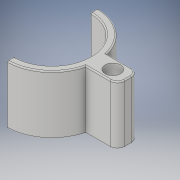
# Autodesk Inventor part: Camera Clip
Saved by Autodesk Inventor 2019.4 (Build 234330000, 330)
## iProperties
Created: 2021-02-04
Part Number: Camera Clip
Material: Generic
Document SubType Name: Modeling
Designer: caleb
Density: 1 g/cm^3
Appearance: Default
Author: caleb
Autodesk Inventor part; units mm, degrees
ref_plane "YZ Plane" through (0, 0, 0) normal (1, 0, 0) x (0, 1, 0)
ref_plane "XZ Plane" through (0, 0, 0) normal (0, 1, 0) x (-1, 0, 0)
ref_plane "XY Plane" through (0, 0, 0) normal (0, 0, 1) x (1, 0, 0)
sketch "Sketch1" plane through (0, 0, 0) normal (0, 1, 0) x (-1, 0, 0)
  circle A0 centre (0, 0) radius 16.51
  circle A1 centre (0, 0) radius 19.685
  line L0 (0, 19.685) -> (0, -19.685)
  line L1 (-32.9172, 4.594) -> (-17.9063, 4.594)
  line L2 (-17.9063, 4.594) -> (-17.9063, -4.594)
  line L3 (-17.9063, -4.594) -> (-32.9172, -4.594)
  line L4 (-32.9172, -4.594) -> (-32.9172, 4.594)
  line L5 (-32.9172, 4.594) -> (-17.9063, -4.594) construction
  line L6 (-17.9063, 4.594) -> (-32.9172, -4.594) construction
  point P0 (-25.4118, 0)
  dimension "d0" = 33.02
  dimension "d1" = 39.37
  constraints: 14 end point, 2 centre point, 2 coincident, 2 midpoint, 2 parallel, 2 point on circle, 1 horizontal, 1 perpendicular, 1 vertical
  measures "d0" diameter of A0
  measures "d1" diameter of A1
extrude "Extrusion1" add sketch "Sketch1" along normal blind 25.4
extrude "Extrusion2" cut sketch "Sketch1" along normal blind 25.4 contours A0 L0 | L0 A0
extrude "Extrusion3" cut sketch "Sketch1" along normal blind 25.4 contours A0 L0 | A0 L0 A1 picked at (8.9586, -4.4939)
sketch "Sketch2" plane through (0, 25.4, 0) normal (0, 1, 0) x (1, 0, 0)
  point P0 (0, 0)
  point P1 (26.3547, 0)
hole "Hole1" at (26.3547, 25.4, 0) direction (0, -1, 0) diameter 6.7564 end through all clearance for "Flat Head Machine Screw (82)" size "1/4" standard "Ansi Unified Screw Threads"
fillet "Fillet1" radius 3.175 2 edges at (32.9172, 12.7, -4.594) (32.9172, 12.7, 4.594)
fillet "Fillet2" radius 0.508 24 edges at (12.1874, 25.4, -15.4585) (16.51, 25.4, 0) (12.1874, 25.4, 15.4585) (0, 12.7, 16.51) (0, 12.7, 19.685) (0, 25.4, 18.0975) (16.51, 0, 0) (12.1874, 0, 15.4585) (0, 0, 18.0975) (0, 0, -18.0975) (0, 12.7, -19.685) (0, 12.7, -16.51) (12.1874, 0, -15.4585) (31.9873, 0, -3.6641) (32.9172, 0, 0) (31.9873, 0, 3.6641) (24.4418, 0, 4.594) (24.4418, 0, -4.594) (31.9873, 25.4, -3.6641) (32.9172, 25.4, 0) (31.9873, 25.4, 3.6641) (24.4418, 25.4, 4.594) (24.4418, 25.4, -4.594) (0, 25.4, -18.0975)
body "Solid1"
